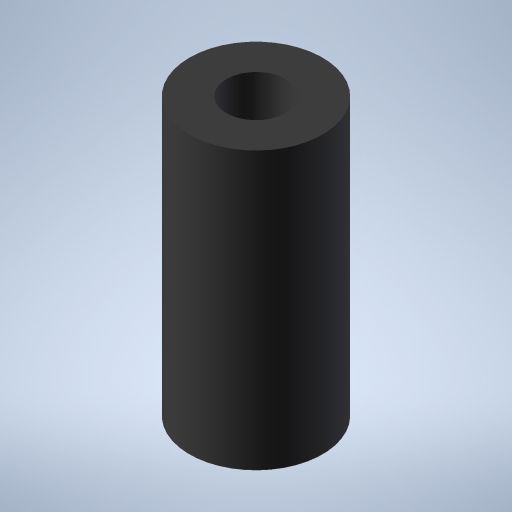
# Autodesk Inventor part: coupler3
Saved by Autodesk Inventor 2023 (Build 270158000, 158)
## iProperties
Created: 2023-02-14
Part Number: coupler3
Material: Generic
Document SubType Name: Modeling
Designer: jxl19
Density: 1 g/cm^3
Appearance: Default
Author: jxl19
## iProperties of the stored document coupler_3DPrint.ipt
Created: 2023-02-14
Part Number: coupler_3DPrint
Material: Generic
Document SubType Name: Modeling
Designer: jxl19
Density: 1 g/cm^3
Appearance: Default
Author: jxl19
Autodesk Inventor part; units mm, degrees
ref_plane "YZ Plane" through (0, 0, 0) normal (1, 0, 0) x (0, 1, 0)
ref_plane "XZ Plane" through (0, 0, 0) normal (0, 1, 0) x (-1, 0, 0)
ref_plane "XY Plane" through (0, 0, 0) normal (0, 0, 1) x (1, 0, 0)
sketch "Sketch1" plane through (0, 0, 0) normal (0, 1, 0) x (-1, 0, 0)
  circle A0 centre (0, 0) radius 2.4
  circle A1 centre (0, 0) radius 0.825
  dimension "d0" = 4.8
  dimension "d1" = 1.65
  constraints: 2 centre point, 2 coincident
  measures "d0" diameter of A0
  measures "d1" diameter of A1
extrude "Extrusion1" add sketch "Sketch1" along normal blind 10
sketch "Sketch2" plane through (0, 10, 0) normal (0, 1, 0) x (1, 0, 0)
  circle A0 centre (0, 0) radius 1.075
  dimension "d4" = 2.15
  constraints: 1 centre point, 1 coincident
  measures "d4" diameter of A0
extrude "Extrusion2" cut sketch "Sketch2" against normal blind 6.2
body "Solid1"
